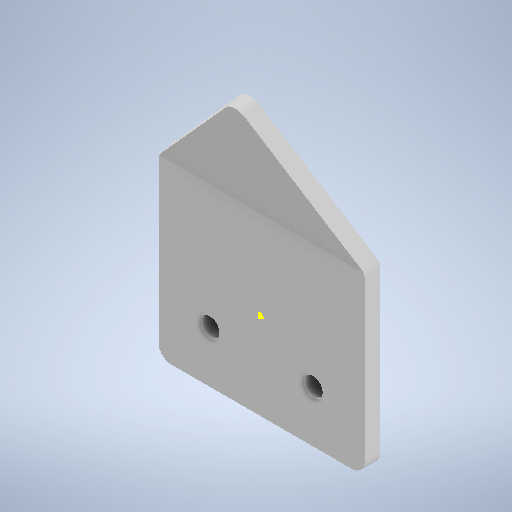
# Autodesk Inventor part: Hook
Saved by Autodesk Inventor 2025.1 (Build 291241020, 241B)
## iProperties
Created: 2024-11-21
Part Number: Hook
Material: Generic
Document SubType Name: Modeling
Designer: AtuStem
Density: 1 g/cm^3
Appearance: Default
Author: AtuStem
Autodesk Inventor part; units mm, degrees
ref_plane "YZ Plane" through (0, 0, 0) normal (1, 0, 0) x (0, 1, 0)
ref_plane "XZ Plane" through (0, 0, 0) normal (0, 1, 0) x (-1, 0, 0)
ref_plane "XY Plane" through (0, 0, 0) normal (0, 0, 1) x (1, 0, 0)
sketch "Sketch1" plane through (0, 0, 0) normal (0, 0, 1) x (1, 0, 0)
  line L0 (-25.4, 21.59) -> (25.4, 21.59)
  line L1 (25.4, 21.59) -> (25.4, -21.59)
  line L2 (25.4, -21.59) -> (-25.4, -21.59)
  line L3 (-25.4, -21.59) -> (-25.4, 21.59)
  line L4 (-25.4, 21.59) -> (25.4, -21.59) construction
  line L5 (25.4, 21.59) -> (-25.4, -21.59) construction
  point P0 (0, 0)
  dimension "d0" = 50.8
  dimension "d18" = 43.18
  constraints: 12 end point, 2 midpoint, 2 parallel, 1 horizontal, 1 perpendicular
  measures "d0" distance of L1.end L2.end
  measures "d18" distance of L2.end L0.start
extrude "Extrusion1" add sketch "Sketch1" along normal blind 3.81
sketch "Sketch2" plane through (25.4, -21.59, 0) normal (1, 0, 0) x (0, 0, -1)
  line L0 (0, 0) -> (0, 43.18) projected
  line L1 (0, 43.18) -> (-7.1849, 71.4926)
  line L2 (-3.81, 43.18) -> (0, 43.18)
  line L3 (-3.81, 43.18) -> (-10.7644, 70.5842)
  line L4 (-10.7644, 70.5842) -> (-7.1849, 71.4926)
  point P0 (0, 21.59)
  dimension "d3" = 29.21
  constraints: 8 end point, 2 perpendicular
  measures "d3" distance of L0.end L1.end
extrude "Extrusion2" add sketch "Sketch2" against normal blind 50.8
sketch "Sketch3" plane through (-25.4, 48.9942, 10.7644) normal (0, -0.2459747, 0.9692762) x (1, 0, 0)
  line L0 (0, 0) -> (0, -29.21) projected
  line L1 (50.8, 0) -> (0, 0) projected
  line L2 (50.8, -29.21) -> (50.8, 0) projected
  line L3 (25.4, 0) -> (50.8, 0)
  line L4 (50.8, 0) -> (50.8, -14.605)
  line L5 (25.4, 0) -> (0, 0)
  line L6 (0, 0) -> (0, -14.605)
  line L7 (50.8, -28.2728) -> (0, -28.2728) projected
  line L8 (0, -28.2728) -> (50.8, -28.2728)
  line L9 (50.8, -28.2728) -> (0, -28.2728)
  line L10 (0, -28.2728) -> (25.4, 0)
  line L11 (25.4, 0) -> (50.8, -28.2728)
  point P0 (25.4, -50.1367)
  constraints: 16 end point, 3 collinear, 3 midpoint, 2 perpendicular, 1 horizontal, 1 point on line
extrude "Extrusion3" cut sketch "Sketch3" against normal blind 72.39 contours L1 L10 L0 | L1 L2 L11
sketch "Sketch5" plane through (0, 0, 3.81) normal (0, 0, 1) x (1, 0, 0)
  line L0 (-25.4, -21.59) -> (25.4, -21.59) projected
  line L1 (-25.4, -21.59) -> (-25.4, -8.89)
  line L2 (-25.4, 21.59) -> (-25.4, -21.59) projected
  line L3 (-25.4, -8.89) -> (-12.7, -8.89)
  line L4 (-12.7, -8.89) -> (12.7, -8.89)
  circle A0 centre (-12.7, -8.89) radius 2.3241
  circle A1 centre (12.7, -8.89) radius 2.3241
  point P0 (0, 0)
  dimension "d11" = 12.7
  dimension "d12" = 12.7
  dimension "d13" = 25.4
  dimension "d14" = 4.6482
  dimension "d15" = 4.6482
  constraints: 6 end point, 2 centre point, 2 coincident, 2 point on line, 1 horizontal
  measures "d11" distance of L0.start L1.end
  measures "d12" distance of L1.end L3.end
  measures "d13" distance of L3.end L4.end
  measures "d14" diameter of A0
  measures "d15" diameter of A1
extrude "Extrusion4" cut sketch "Sketch5" against normal blind 50.8
fillet "Fillet1" radius 3.175 1 edges at (0, 49.4484, 8.9747)
fillet "Fillet2" radius 3.175 4 edges at (25.4, -21.59, 1.905) (-25.4, -21.59, 1.905) (-25.4, 22.0442, 2.0203) (25.4, 22.0442, 2.0203)
sketch "Sketch6" plane through (0, 0, 3.81) normal (0, 0, 1) x (1, 0, 0)
  point P0 (0, 0)
body "Solid1"
